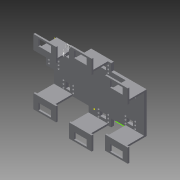
# Autodesk Inventor part: BassStuffMounts
Saved by Autodesk Inventor 2015 (Build 190159000, 159)
## iProperties
Created: 2016-04-25
Part Number: BassStuffMounts
Material: Generic
Document SubType Name: Modeling
Designer: Hatch
Density: 1 g/cm^3
Appearance: Default
Author: Hatch
Autodesk Inventor part; units mm, degrees
ref_plane "YZ Plane" through (0, 0, 0) normal (1, 0, 0) x (0, 1, 0)
ref_plane "XZ Plane" through (0, 0, 0) normal (0, 1, 0) x (-1, 0, 0)
ref_plane "XY Plane" through (0, 0, 0) normal (0, 0, 1) x (1, 0, 0)
sketch "Sketch1" plane through (0, 0, 0) normal (0, 1, 0) x (-1, 0, 0)
  line L0 (-75, 37.5) -> (75, 37.5)
  line L1 (75, 37.5) -> (75, -37.5)
  line L2 (75, -37.5) -> (-75, -37.5)
  line L3 (-75, -37.5) -> (-75, 37.5)
  line L4 (-75, 37.5) -> (75, -37.5) construction
  line L5 (75, 37.5) -> (-75, -37.5) construction
  point P0 (0, 0)
  dimension "d0" = 150
  dimension "d1" = 75
  constraints: 12 end point, 2 midpoint, 2 parallel, 1 horizontal, 1 perpendicular
  measures "d0" distance of L1.end L2.end
  measures "d1" distance of L0.end L1.end
extrude "Extrusion1" add sketch "Sketch1" along normal blind 5
sketch "Sketch2" plane through (0, 5, 0) normal (0, 1, 0) x (1, 0, 0)
  point P0 (0, 0)
sketch "Sketch3" plane through (0, 5, 0) normal (0, 1, 0) x (1, 0, 0)
  line L0 (75, 37.5) -> (-75, 37.5) projected
  line L1 (-75, 37.5) -> (-75, -37.5) projected
  line L2 (-75, 0) -> (75, 0)
  line L3 (75, -37.5) -> (75, 37.5) projected
  line L4 (-75, 0) -> (-75, -37.5)
  line L5 (-75, 0) -> (-75, 37.5)
  line L6 (-75, -18.75) -> (75, -18.75)
  line L7 (-75, 18.75) -> (75, 18.75)
  line L8 (-75, -37.5) -> (75, -37.5)
  line L9 (-75, -37.5) -> (75, -37.5) projected
  line L10 (-75, -37.5) -> (-25, -37.5)
  line L11 (-25, -37.5) -> (25, -37.5)
  line L12 (25, -37.5) -> (75, -37.5)
  line L13 (25, -37.5) -> (25, 37.5)
  line L14 (-25, -37.5) -> (-25, 37.5)
  line L15 (-75, 37.5) -> (-39, 37.5)
  line L16 (-39, 37.5) -> (-39, 13.5)
  line L17 (-39, 13.5) -> (-75, 13.5)
  line L18 (-75, 13.5) -> (-75, 37.5)
  line L19 (-75, -37.5) -> (-39, -37.5)
  line L20 (-39, -37.5) -> (-39, -13.5)
  line L21 (-39, -13.5) -> (-75, -13.5)
  line L22 (-75, -13.5) -> (-75, -37.5)
  line L23 (-67.8885, -37.5) -> (-67.8885, -31.5)
  line L24 (-70.151, 37.5) -> (-70.151, 31.5)
  line L25 (-75, -23.3322) -> (-67, -23.3322)
  circle A0 centre (-67, -31.5) radius 2.125
  line L26 (-67, -31.5) -> (-49, -31.5)
  circle A1 centre (-49, -31.5) radius 2.125
  line L27 (-67, -31.5) -> (-67, -25.5)
  line L28 (-67, -25.5) -> (-67, -19.5)
  circle A2 centre (-67, -25.5) radius 2.125
  circle A3 centre (-67, -19.5) radius 2.125
  line L29 (-49, -31.5) -> (-49, -25.5)
  line L30 (-49, -25.5) -> (-49, -19.5)
  circle A4 centre (-49, -25.5) radius 2.125
  circle A5 centre (-49, -19.5) radius 2.125
  circle A6 centre (-67, 31.5) radius 2.125
  line L31 (-67, 31.5) -> (-67, 25.5)
  line L32 (-67, 25.5) -> (-67, 19.5)
  line L33 (-67, 19.5) -> (-49, 19.5)
  line L34 (-49, 19.5) -> (-49, 25.5)
  line L35 (-49, 25.5) -> (-49, 31.5)
  circle A7 centre (-49, 31.5) radius 2.125
  circle A8 centre (-49, 25.5) radius 2.125
  circle A9 centre (-49, 19.5) radius 2.125
  circle A10 centre (-67, 25.5) radius 2.125
  circle A11 centre (-67, 19.5) radius 2.125
  point P0 (0, 0)
  dimension "d4" = 50
  dimension "d5" = 50
  dimension "d6" = 50
  dimension "d7" = 36
  dimension "d8" = 24
  dimension "d10" = 36
  dimension "d11" = 24
  dimension "d12" = 6
  dimension "d13" = 6
  dimension "d17" = 8
  dimension "d18" = 4.25
  dimension "d19" = 18
  dimension "d20" = 4.25
  dimension "d21" = 6
  dimension "d22" = 6
  dimension "d23" = 4.25
  dimension "d24" = 4.25
  dimension "d25" = 6
  dimension "d26" = 6
  dimension "d27" = 4.25
  dimension "d28" = 4.25
  dimension "d29" = 4.25
  dimension "d30" = 6
  dimension "d31" = 6
  dimension "d32" = 18
  dimension "d33" = 6
  dimension "d34" = 6
  dimension "d35" = 4.25
  dimension "d36" = 4.25
  dimension "d37" = 4.25
  dimension "d38" = 4.25
  dimension "d39" = 4.25
  constraints: 64 end point, 13 point on line, 12 centre point, 10 coincident, 10 perpendicular, 5 parallel, 4 collinear, 4 midpoint, 3 horizontal, 3 vertical
  measures "d4" distance of L1.end L10.end
  measures "d5" distance of L10.end L11.end
  measures "d6" distance of L11.end L3.start
  measures "d7" distance of L16.end L17.end
  measures "d8" distance of L15.end L16.end
  measures "d10" distance of L21.end L20.end
  measures "d11" distance of L20.end L19.end
  measures "d12" distance of L23.start L23.end
  measures "d13" distance of L24.start L24.end
  measures "d17" distance of L25.start L25.end
  measures "d18" diameter of A0
  measures "d19" distance of L26.start L26.end
  measures "d20" diameter of A1
  measures "d21" distance of L26.start L27.end
  measures "d22" distance of L27.end L28.end
  measures "d23" diameter of A2
  measures "d24" diameter of A3
  measures "d25" distance of L29.start L29.end
  measures "d26" distance of L29.end L30.end
  measures "d27" diameter of A4
  measures "d28" diameter of A5
  measures "d29" diameter of A6
  measures "d30" distance of L31.start L31.end
  measures "d31" distance of L31.end L32.end
  measures "d32" distance of L32.end L33.end
  measures "d33" distance of L33.end L34.end
  measures "d34" distance of L34.end L35.end
  measures "d35" diameter of A7
  measures "d36" diameter of A8
  measures "d37" diameter of A9
  measures "d38" diameter of A10
  measures "d39" diameter of A11
sketch "Sketch4" plane through (0, 0, 0) normal (0, -1, 0) x (1, 0, 0)
  line L0 (-75, -37.5) -> (-41, -37.5)
  line L1 (-41, -37.5) -> (-41, -34.5)
  line L2 (-41, -34.5) -> (-75, -34.5)
  line L3 (-75, -34.5) -> (-75, -37.5)
  circle A0 centre (-49, -25.5) radius 2.125 projected
  line L4 (-75, 37.5) -> (-41, 37.5)
  line L5 (-41, 37.5) -> (-41, 34.5)
  line L6 (-41, 34.5) -> (-75, 34.5)
  line L7 (-75, 34.5) -> (-75, 37.5)
  point P0 (0, 0)
  dimension "d42" = 34
  dimension "d43" = 3
  dimension "d45" = 3
  constraints: 16 end point, 4 parallel, 2 horizontal, 2 perpendicular
  measures "d42" distance of L2.end L1.end
  measures "d43" distance of L1.end L0.end
  measures "d45" distance of L4.end L5.end
extrude "Extrusion3" add sketch "Sketch4" along normal blind 34.05 contours L3 L2 L1 L0 | L4 L5 L6 L7
sketch "Sketch5" plane through (0, -34.05, 0) normal (0, -1, 0) x (1, 0, 0)
  line L0 (-75, -34.5) -> (-79, -34.5)
  line L1 (-79, -34.5) -> (-79, -37.5)
  line L2 (-79, -37.5) -> (-75, -37.5)
  line L3 (-75, -37.5) -> (-75, -34.5)
  line L4 (-41, -37.5) -> (-37, -37.5)
  line L5 (-37, -37.5) -> (-37, -34.5)
  line L6 (-37, -34.5) -> (-41, -34.5)
  line L7 (-41, -34.5) -> (-41, -37.5)
  line L8 (-75, 37.5) -> (-79, 37.5)
  line L9 (-79, 37.5) -> (-79, 34.5)
  line L10 (-79, 34.5) -> (-75, 34.5)
  line L11 (-75, 34.5) -> (-75, 37.5)
  line L12 (-41, 34.5) -> (-37, 34.5)
  line L13 (-37, 34.5) -> (-37, 37.5)
  line L14 (-37, 37.5) -> (-41, 37.5)
  line L15 (-41, 37.5) -> (-41, 34.5)
  point P0 (0, 0)
  dimension "d48" = 4
  dimension "d49" = 3
  dimension "d50" = 4
  dimension "d51" = 3
  dimension "d52" = 4
  dimension "d53" = 3
  dimension "d54" = 4
  dimension "d55" = 3
  constraints: 32 end point, 8 parallel, 4 horizontal, 4 perpendicular
  measures "d48" distance of L2.end L1.end
  measures "d49" distance of L1.end L0.end
  measures "d50" distance of L6.end L5.end
  measures "d51" distance of L5.end L4.end
  measures "d52" distance of L10.end L9.end
  measures "d53" distance of L9.end L8.end
  measures "d54" distance of L14.end L13.end
  measures "d55" distance of L13.end L12.end
extrude "Extrusion4" add sketch "Sketch5" against normal blind 3
sketch "Sketch6" plane through (-75, 5, 37.5) normal (0, 0, 1) x (1, 0, 0)
  line L0 (38, -39.05) -> (-4, -39.05)
  line L1 (-4, -39.05) -> (-4, -36.05)
  line L2 (-4, -36.05) -> (38, -36.05)
  line L3 (38, -36.05) -> (38, -39.05)
  point P0 (75, -5)
  constraints: 8 end point, 2 parallel, 1 horizontal, 1 perpendicular
extrude "Extrusion5" add sketch "Sketch6" along normal blind 23
sketch "Sketch7" plane through (75, 5, -37.5) normal (0, 0, -1) x (-1, 0, 0)
  line L0 (154, -39.05) -> (112, -39.05)
  line L1 (112, -39.05) -> (112, -36.05)
  line L2 (112, -36.05) -> (154, -36.05)
  line L3 (154, -36.05) -> (154, -39.05)
  point P0 (75, -5)
  constraints: 8 end point, 2 parallel, 1 horizontal, 1 perpendicular
extrude "Extrusion6" add sketch "Sketch7" along normal blind 23
sketch "Sketch9" plane through (0, 5, 0) normal (0, 1, 0) x (1, 0, 0)
  line L0 (-79, 60.5) -> (-37, 60.5)
  line L1 (-79, 60.5) -> (-37, 60.5) projected
  line L2 (75, 37.5) -> (-75, 37.5) projected
  line L3 (-58, 37.5) -> (-58, 31.5)
  circle A0 centre (-58, 31.5) radius 2.125
  line L4 (-58, 31.5) -> (-40, 31.5)
  line L5 (-40, 31.5) -> (-40, 25.5)
  line L6 (-40, 25.5) -> (-40, 19.5)
  circle A1 centre (-40, 31.5) radius 2.125
  circle A2 centre (-40, 25.5) radius 2.125
  circle A3 centre (-40, 19.5) radius 2.125
  circle A4 centre (-58, 25.5) radius 2.125
  circle A5 centre (-58, 19.5) radius 2.125
  line L7 (-79, -60.5) -> (-37, -60.5)
  line L8 (-79, -60.5) -> (-37, -60.5) projected
  line L9 (-75, -37.5) -> (75, -37.5) projected
  line L10 (-58, -37.5) -> (-58, -31.5)
  circle A6 centre (-58, -31.5) radius 2.125
  line L11 (-58, -31.5) -> (-40, -31.5)
  line L12 (-40, -31.5) -> (-40, -25.5)
  line L13 (-40, -25.5) -> (-40, -19.5)
  circle A7 centre (-40, -31.5) radius 2.125
  circle A8 centre (-40, -25.5) radius 2.125
  circle A9 centre (-40, -19.5) radius 2.125
  circle A10 centre (-58, -25.5) radius 2.125
  circle A11 centre (-58, -19.5) radius 2.125
  point P0 (0, 0)
  dimension "d62" = 6
  dimension "d63" = 4.25
  dimension "d64" = 18
  dimension "d65" = 6
  dimension "d66" = 6
  dimension "d67" = 4.25
  dimension "d68" = 4.25
  dimension "d69" = 4.25
  dimension "d70" = 4.25
  dimension "d71" = 4.25
  dimension "d72" = 6
  dimension "d73" = 4.25
  dimension "d74" = 18
  dimension "d75" = 6
  dimension "d76" = 6
  dimension "d77" = 4.25
  dimension "d78" = 4.25
  dimension "d79" = 4.25
  dimension "d80" = 4.25
  dimension "d81" = 4.25
  constraints: 20 end point, 12 centre point, 8 coincident, 4 horizontal, 3 point on line, 2 perpendicular, 1 vertical
  measures "d62" distance of L3.start L3.end
  measures "d63" diameter of A0
  measures "d64" distance of L4.start L4.end
  measures "d65" distance of L4.end L5.end
  measures "d66" distance of L5.end L6.end
  measures "d67" diameter of A1
  measures "d68" diameter of A2
  measures "d69" diameter of A3
  measures "d70" diameter of A4
  measures "d71" diameter of A5
  measures "d72" distance of L10.start L10.end
  measures "d73" diameter of A6
  measures "d74" distance of L11.start L11.end
  measures "d75" distance of L11.end L12.end
  measures "d76" distance of L12.end L13.end
  measures "d77" diameter of A7
  measures "d78" diameter of A8
  measures "d79" diameter of A9
  measures "d80" diameter of A10
  measures "d81" diameter of A11
extrude "Extrusion7" cut sketch "Sketch9" against normal through all
sketch "Sketch10" plane through (0, -34.05, 0) normal (0, -1, 0) x (1, 0, 0)
  line L0 (-75, -34.5) -> (-41, -34.5) projected
  line L1 (-58, -34.5) -> (-58, -45.5)
  line L2 (-41, 34.5) -> (-75, 34.5) projected
  line L3 (-58, 34.5) -> (-58, 45.5)
  line L4 (-37, -60.5) -> (-37, -34.5) projected
  line L5 (-37, -47.5) -> (-39.25, -47.5)
  line L6 (-79, -34.5) -> (-79, -60.5) projected
  line L7 (-79, -47.5) -> (-76.75, -47.5)
  line L8 (-79, -60.5) -> (-37, -60.5) projected
  line L9 (-58, -60.5) -> (-58, -57.5)
  line L10 (-46.25, -57.5) -> (-69.75, -57.5)
  line L11 (-69.75, -57.5) -> (-69.75, -45.5)
  line L12 (-69.75, -45.5) -> (-46.25, -45.5)
  line L13 (-46.25, -45.5) -> (-46.25, -57.5)
  line L14 (-79, 34.5) -> (-79, 60.5) projected
  line L15 (-79, 47.5) -> (-76.75, 47.5)
  line L16 (-37, 34.5) -> (-37, 60.5) projected
  line L17 (-37, 47.5) -> (-39.25, 47.5)
  line L18 (-37, 60.5) -> (-79, 60.5) projected
  line L19 (-58, 60.5) -> (-58, 57.5)
  line L20 (-46.25, 57.5) -> (-69.75, 57.5)
  line L21 (-69.75, 57.5) -> (-69.75, 45.5)
  line L22 (-69.75, 45.5) -> (-46.25, 45.5)
  line L23 (-46.25, 45.5) -> (-46.25, 57.5)
  point P0 (0, 0)
  dimension "d84" = 11
  dimension "d85" = 11
  dimension "d86" = 2.25
  dimension "d87" = 2.25
  dimension "d88" = 3
  dimension "d89" = 2.25
  dimension "d90" = 2.25
  dimension "d91" = 3
  dimension "d115" = 23.5
  dimension "d116" = 23.5
  constraints: 32 end point, 10 midpoint, 6 horizontal, 4 parallel, 4 vertical, 2 perpendicular
  measures "d84" distance of L1.start L1.end
  measures "d85" distance of L3.end L3.start
  measures "d86" distance of L5.start L5.end
  measures "d87" distance of L7.start L7.end
  measures "d88" distance of L9.end L9.start
  measures "d89" distance of L15.start L15.end
  measures "d90" distance of L17.start L17.end
  measures "d91" distance of L19.start L19.end
  measures "d115" distance of L10.start L10.end
  measures "d116" distance of L20.start L20.end
extrude "Extrusion8" cut sketch "Sketch10" against normal through all
sketch "Sketch14" plane through (0, 5, 0) normal (0, 1, 0) x (1, 0, 0)
  line L0 (-75, -37.5) -> (75, -37.5) projected
  line L1 (75, 37.5) -> (-32.8207, 37.5)
  line L2 (-32.8207, 37.5) -> (-32.8207, -37.5)
  line L3 (-32.8207, -37.5) -> (75, -37.5)
  line L4 (75, -37.5) -> (75, 37.5)
  point P0 (0, 0)
  constraints: 8 end point, 2 parallel, 1 horizontal, 1 perpendicular, 1 point on line
sketch "Sketch15" plane through (0, 0, 0) normal (0, -1, 0) x (1, 0, 0)
  circle A0 centre (-40, 25.5) radius 2.125 projected
  line L0 (-40, 25.5) -> (-49, 25.5)
  line L1 (-53, 20) -> (-45, 20)
  line L2 (-45, 20) -> (-45, 31)
  line L3 (-45, 31) -> (-53, 31)
  line L4 (-53, 31) -> (-53, 20)
  line L5 (-53, 20) -> (-45, 31) construction
  line L6 (-45, 20) -> (-53, 31) construction
  line L7 (-53, -31) -> (-45, -31)
  line L8 (-45, -31) -> (-45, -20)
  line L9 (-45, -20) -> (-53, -20)
  line L10 (-53, -20) -> (-53, -31)
  line L11 (-53, -31) -> (-45, -20) construction
  line L12 (-45, -31) -> (-53, -20) construction
  point P0 (0, 0)
  point P1 (-49, -25.5)
  dimension "d108" = 9
  dimension "d109" = 8
  dimension "d110" = 11
  dimension "d111" = 8
  dimension "d112" = 11
  constraints: 26 end point, 4 midpoint, 4 parallel, 3 horizontal, 2 perpendicular
  measures "d108" distance of L0.start L0.end
  measures "d109" distance of L3.end L2.end
  measures "d110" distance of L2.end L1.end
  measures "d111" distance of L9.end L8.end
  measures "d112" distance of L8.end L7.end
extrude "Extrusion13" cut sketch "Sketch15" against normal through all contours L4 L3 L2 L1 | L10 L9 L8 L7
sketch "Sketch16" plane through (0, -34.05, 0) normal (0, -1, 0) x (1, 0, 0)
  point P0 (0, 0)
sketch "Sketch18" plane through (0, 5, 0) normal (0, 1, 0) x (1, 0, 0)
  point P0 (0, 0)
sketch "Sketch19" plane through (0, 5, 0) normal (0, 1, 0) x (1, 0, 0)
  line L0 (-75, -37.5) -> (75, -37.5) projected
  line L1 (25.0535, -37.5) -> (-10.9465, -37.5)
  line L2 (-10.9465, -37.5) -> (-10.9465, -13.5)
  line L3 (-10.9465, -13.5) -> (25.0535, -13.5)
  line L4 (25.0535, -13.5) -> (25.0535, -37.5)
  line L5 (-41, 37.5) -> (75, 37.5) projected
  line L6 (25.0535, 37.5) -> (-10.9465, 37.5)
  line L7 (-10.9465, 37.5) -> (-10.9465, 13.5)
  line L8 (-10.9465, 13.5) -> (25.0535, 13.5)
  line L9 (25.0535, 13.5) -> (25.0535, 37.5)
  line L10 (-10.9465, 37.5) -> (25.0535, 37.5)
  line L11 (25.0535, 37.5) -> (25.0535, 51.5)
  line L12 (25.0535, 51.5) -> (-10.9465, 51.5)
  line L13 (-10.9465, 51.5) -> (-10.9465, 37.5)
  line L14 (-10.9465, -37.5) -> (25.0535, -37.5)
  line L15 (25.0535, -37.5) -> (25.0535, -51.5)
  line L16 (25.0535, -51.5) -> (-10.9465, -51.5)
  line L17 (-10.9465, -51.5) -> (-10.9465, -37.5)
  point P0 (0, 0)
  dimension "d117" = 36
  dimension "d118" = 24
  dimension "d119" = 36
  dimension "d120" = 24
  dimension "d121" = 14
  dimension "d122" = 14
  constraints: 32 end point, 8 parallel, 4 horizontal, 4 perpendicular, 4 point on line
  measures "d117" distance of L2.end L3.end
  measures "d118" distance of L1.end L2.end
  measures "d119" distance of L8.end L7.end
  measures "d120" distance of L7.end L6.end
  measures "d121" distance of L11.end L10.end
  measures "d122" distance of L14.end L15.end
extrude "Extrusion14" add sketch "Sketch19" against normal blind 5 contours L0 L15 L16 L17 | L13 L12 L11 L5
sketch "Sketch21" plane through (0, 0, 0) normal (0, -1, 0) x (1, 0, 0)
  line L0 (-10.9465, -37.5) -> (-10.9465, -51.5) projected
  line L1 (25.0535, -51.5) -> (-10.9465, -51.5)
  line L2 (-10.9465, -51.5) -> (-10.9465, -48.5)
  line L3 (-10.9465, -48.5) -> (25.0535, -48.5)
  line L4 (25.0535, -48.5) -> (25.0535, -51.5)
  line L5 (25.0535, 37.5) -> (25.0535, 51.5) projected
  line L6 (-10.9465, 51.5) -> (25.0535, 51.5)
  line L7 (25.0535, 51.5) -> (25.0535, 48.5)
  line L8 (25.0535, 48.5) -> (-10.9465, 48.5)
  line L9 (-10.9465, 48.5) -> (-10.9465, 51.5)
  point P0 (0, 0)
  dimension "d153" = 3
  dimension "d154" = 3
  constraints: 16 end point, 4 parallel, 2 horizontal, 2 perpendicular, 2 point on line
  measures "d153" distance of L1.end L2.end
  measures "d154" distance of L6.end L7.end
extrude "Extrusion16" add sketch "Sketch21" along normal blind 34.05
sketch "Sketch23" plane through (0, -34.05, 0) normal (0, -1, 0) x (1, 0, 0)
  line L0 (25.0535, 48.5) -> (29.0535, 48.5)
  line L1 (25.0535, -48.5) -> (29.0535, -48.5)
  line L2 (29.0535, 48.5) -> (-12.9465, 48.5)
  line L3 (-12.9465, 48.5) -> (-12.9465, 74.5)
  line L4 (-12.9465, 74.5) -> (29.0535, 74.5)
  line L5 (29.0535, 74.5) -> (29.0535, 48.5)
  line L6 (29.0535, -48.5) -> (-12.9465, -48.5)
  line L7 (-12.9465, -48.5) -> (-12.9465, -74.5)
  line L8 (-12.9465, -74.5) -> (29.0535, -74.5)
  line L9 (29.0535, -74.5) -> (29.0535, -48.5)
  point P0 (0, 0)
  dimension "d157" = 4
  dimension "d158" = 42
  dimension "d159" = 26
  dimension "d160" = 26
  constraints: 20 end point, 4 horizontal, 4 parallel, 2 perpendicular
  measures "d157" distance of L0.start L0.end
  measures "d158" distance of L3.end L4.end
  measures "d159" distance of L2.end L3.end
  measures "d160" distance of L7.end L6.end
extrude "Extrusion17" add sketch "Sketch23" against normal blind 3
sketch "Sketch24" plane through (0, 5, 0) normal (0, 1, 0) x (1, 0, 0)
  line L0 (25.0535, -37.5) -> (31.0535, -37.5)
  line L1 (31.0535, -37.5) -> (31.0535, -51.5)
  line L2 (31.0535, -51.5) -> (25.0535, -51.5)
  line L3 (25.0535, -51.5) -> (25.0535, -37.5)
  line L4 (25.0535, 51.5) -> (31.0535, 51.5)
  line L5 (31.0535, 51.5) -> (31.0535, 37.5)
  line L6 (31.0535, 37.5) -> (25.0535, 37.5)
  line L7 (25.0535, 37.5) -> (25.0535, 51.5)
  point P0 (0, 0)
  dimension "d169" = 6
  dimension "d170" = 6
  constraints: 16 end point, 4 parallel, 2 horizontal, 2 perpendicular
  measures "d169" distance of L1.end L2.end
  measures "d170" distance of L5.end L6.end
extrude "Extrusion18" add sketch "Sketch24" against normal blind 5
sketch "Sketch20" plane through (0, 5, 0) normal (0, 1, 0) x (1, 0, 0)
  line L0 (25.0535, -51.5) -> (-10.9465, -51.5) projected
  line L1 (7.0535, -51.5) -> (7.0535, -45.5)
  line L2 (7.0535, -45.5) -> (16.0535, -45.5)
  line L3 (16.0535, -45.5) -> (-1.9465, -45.5)
  line L4 (-10.9465, 51.5) -> (25.0535, 51.5) projected
  line L5 (25.0535, 51.5) -> (-10.9465, 51.5) projected
  line L6 (-6.3335, 51.5) -> (-6.3335, 45.5)
  line L7 (16.0535, -45.5) -> (16.0535, -39.5)
  line L8 (16.0535, -39.5) -> (16.0535, -33.5)
  circle A0 centre (7.0535, 39.5) radius 2.125
  circle A1 centre (7.0535, 45.5) radius 2.125
  circle A2 centre (7.0535, 33.5) radius 2.125
  circle A3 centre (7.0535, -33.5) radius 2.125
  circle A4 centre (7.0535, -39.5) radius 2.125
  circle A5 centre (7.0535, -45.5) radius 2.125
  line L9 (7.0535, -33.5) -> (25.0535, -33.5)
  circle A6 centre (25.0535, -33.5) radius 2.125
  circle A7 centre (25.0535, -39.5) radius 2.125
  circle A8 centre (25.0535, -45.5) radius 2.125
  circle A9 centre (25.0535, 45.5) radius 2.125
  circle A10 centre (25.0535, 39.5) radius 2.125
  circle A11 centre (25.0535, 33.5) radius 2.125
  line L10 (21.5535, -43.5) -> (10.5535, -43.5)
  line L11 (10.5535, -43.5) -> (10.5535, -35.5)
  line L12 (10.5535, -35.5) -> (21.5535, -35.5)
  line L13 (21.5535, -35.5) -> (21.5535, -43.5)
  line L14 (21.5535, -43.5) -> (10.5535, -35.5) construction
  line L15 (10.5535, -43.5) -> (21.5535, -35.5) construction
  line L16 (21.5535, 35.5) -> (10.5535, 35.5)
  line L17 (10.5535, 35.5) -> (10.5535, 43.5)
  line L18 (10.5535, 43.5) -> (21.5535, 43.5)
  line L19 (21.5535, 43.5) -> (21.5535, 35.5)
  line L20 (21.5535, 35.5) -> (10.5535, 43.5) construction
  line L21 (10.5535, 35.5) -> (21.5535, 43.5) construction
  point P0 (0, 0)
  point P1 (16.0535, 39.5)
  dimension "d125" = 6
  dimension "d126" = 9
  dimension "d127" = 18
  dimension "d130" = 6
  dimension "d135" = 6
  dimension "d136" = 6
  dimension "d164" = 4.25
  dimension "d165" = 4.25
  dimension "d166" = 4.25
  dimension "d167" = 4.25
  dimension "d168" = 4.25
  dimension "d173" = 4.25
  dimension "d174" = 4.25
  dimension "d175" = 4.25
  dimension "d176" = 4.25
  dimension "d177" = 4.25
  dimension "d178" = 4.25
  dimension "d179" = 11
  dimension "d180" = 8
  dimension "d181" = 11
  dimension "d182" = 8
  constraints: 38 end point, 12 centre point, 5 midpoint, 5 perpendicular, 4 coincident, 4 parallel, 4 point on line, 3 horizontal, 1 vertical
  measures "d125" distance of L1.start L1.end
  measures "d126" distance of L1.end L2.end
  measures "d127" distance of L2.end L3.end
  measures "d130" distance of L6.start L6.end
  measures "d135" distance of L2.end L7.end
  measures "d136" distance of L7.end L8.end
  measures "d164" diameter of A1
  measures "d165" diameter of A2
  measures "d166" diameter of A3
  measures "d167" diameter of A4
  measures "d168" diameter of A5
  measures "d173" diameter of A6
  measures "d174" diameter of A7
  measures "d175" diameter of A8
  measures "d176" diameter of A9
  measures "d177" diameter of A10
  measures "d178" diameter of A11
  measures "d179" distance of L11.end L12.end
  measures "d180" distance of L10.end L11.end
  measures "d181" distance of L17.end L18.end
  measures "d182" distance of L16.end L17.end
extrude "Extrusion19" cut sketch "Sketch20" against normal through all
sketch "Sketch25" plane through (0, -34.05, 0) normal (0, -1, 0) x (1, 0, 0)
  line L0 (29.0535, -74.5) -> (-12.9465, -74.5) projected
  line L1 (8.0535, -74.5) -> (8.0535, -71.5)
  line L2 (-12.9465, 74.5) -> (29.0535, 74.5) projected
  line L3 (8.0535, 74.5) -> (8.0535, 71.5)
  line L4 (8.0535, -71.5) -> (8.0535, -59.5)
  line L5 (8.0535, 71.5) -> (8.0535, 59.5)
  line L6 (19.8035, 71.5) -> (-3.6965, 71.5)
  line L7 (-3.6965, 71.5) -> (-3.6965, 59.5)
  line L8 (-3.6965, 59.5) -> (19.8035, 59.5)
  line L9 (19.8035, 59.5) -> (19.8035, 71.5)
  line L10 (19.8035, 71.5) -> (-3.6965, 59.5) construction
  line L11 (-3.6965, 71.5) -> (19.8035, 59.5) construction
  line L12 (19.8035, -59.5) -> (-3.6965, -59.5)
  line L13 (-3.6965, -59.5) -> (-3.6965, -71.5)
  line L14 (-3.6965, -71.5) -> (19.8035, -71.5)
  line L15 (19.8035, -71.5) -> (19.8035, -59.5)
  line L16 (19.8035, -59.5) -> (-3.6965, -71.5) construction
  line L17 (-3.6965, -59.5) -> (19.8035, -71.5) construction
  point P0 (0, 0)
  point P1 (8.0535, 65.5)
  point P2 (8.0535, -65.5)
  dimension "d185" = 3
  dimension "d186" = 3
  dimension "d187" = 12
  dimension "d188" = 12
  dimension "d189" = 23.5
  dimension "d190" = 23.5
  constraints: 32 end point, 8 midpoint, 4 parallel, 4 vertical, 2 horizontal, 2 perpendicular
  measures "d185" distance of L1.start L1.end
  measures "d186" distance of L3.start L3.end
  measures "d187" distance of L1.end L4.end
  measures "d188" distance of L3.end L5.end
  measures "d189" distance of L8.end L7.end
  measures "d190" distance of L14.end L13.end
extrude "Extrusion20" cut sketch "Sketch25" against normal through all
sketch "Sketch27" plane through (0, -34.05, 0) normal (0, -1, 0) x (1, 0, 0)
  line L0 (-46.25, -57.5) -> (-69.75, -57.5) projected
  line L1 (-58, -57.5) -> (8.0535, -57.5)
  line L2 (-3.6965, -59.5) -> (19.8035, -59.5) projected
  line L3 (8.0535, -57.5) -> (74.1075, -57.5)
  point P0 (0, 0)
  dimension "d193" = 66.0535
  dimension "d194" = 66.054
  constraints: 4 end point, 1 horizontal, 1 midpoint, 1 parallel
  measures "d193" distance of L1.start L1.end
  measures "d194" distance of L1.end L3.end
sketch "Sketch28" plane through (0, 0, 0) normal (0, -1, 0) x (1, 0, 0)
  circle A0 centre (-40, -31.5) radius 2.125 projected
  line L0 (75, 37.5) -> (75, -37.5) projected
  circle A1 centre (75, -31.5) radius 2.125
  line L1 (75, -31.5) -> (57, -31.5)
  circle A2 centre (57, -31.5) radius 2.125
  line L2 (57, -31.5) -> (57, -25.5)
  line L3 (57, -25.5) -> (57, -19.5)
  circle A3 centre (57, -25.5) radius 2.125
  circle A4 centre (57, -19.5) radius 2.125
  circle A5 centre (75, -25.5) radius 2.125
  circle A6 centre (75, -19.5) radius 2.125
  circle A7 centre (-40, 31.5) radius 2.125 projected
  line L4 (-40, 31.5) -> (75, 31.5)
  circle A8 centre (75, 31.5) radius 2.125
  line L5 (75, 31.5) -> (57, 31.5)
  line L6 (57, 31.5) -> (57, 25.5)
  line L7 (57, 25.5) -> (57, 19.5)
  circle A9 centre (57, 31.5) radius 2.125
  circle A10 centre (57, 25.5) radius 2.125
  circle A11 centre (57, 19.5) radius 2.125
  circle A12 centre (75, 25.5) radius 2.125
  circle A13 centre (75, 19.5) radius 2.125
  line L8 (71.5, -29.5) -> (60.5, -29.5)
  line L9 (60.5, -29.5) -> (60.5, -21.5)
  line L10 (60.5, -21.5) -> (71.5, -21.5)
  line L11 (71.5, -21.5) -> (71.5, -29.5)
  line L12 (71.5, -29.5) -> (60.5, -21.5) construction
  line L13 (60.5, -29.5) -> (71.5, -21.5) construction
  line L14 (71.5, 21.5) -> (60.5, 21.5)
  line L15 (60.5, 21.5) -> (60.5, 29.5)
  line L16 (60.5, 29.5) -> (71.5, 29.5)
  line L17 (71.5, 29.5) -> (71.5, 21.5)
  line L18 (71.5, 21.5) -> (60.5, 29.5) construction
  line L19 (60.5, 21.5) -> (71.5, 29.5) construction
  point P0 (0, 0)
  point P1 (66, -25.5)
  point P2 (66, 25.5)
  dimension "d195" = 4.25
  dimension "d196" = 18
  dimension "d197" = 4.25
  dimension "d198" = 6
  dimension "d199" = 6
  dimension "d200" = 4.25
  dimension "d201" = 4.25
  dimension "d202" = 4.25
  dimension "d203" = 4.25
  dimension "d204" = 4.25
  dimension "d205" = 6
  dimension "d206" = 6
  dimension "d207" = 4.25
  dimension "d208" = 4.25
  dimension "d209" = 4.25
  dimension "d210" = 4.25
  dimension "d211" = 4.25
  dimension "d212" = 11
  dimension "d213" = 8
  dimension "d214" = 11
  dimension "d215" = 8
  constraints: 38 end point, 12 centre point, 8 point on line, 7 coincident, 4 midpoint, 4 parallel, 4 perpendicular, 3 horizontal, 1 vertical
  measures "d195" diameter of A1
  measures "d196" distance of L1.start L1.end
  measures "d197" diameter of A2
  measures "d198" distance of L2.start L2.end
  measures "d199" distance of L2.end L3.end
  measures "d200" diameter of A3
  measures "d201" diameter of A4
  measures "d202" diameter of A5
  measures "d203" diameter of A6
  measures "d204" diameter of A8
  measures "d205" distance of L5.end L6.end
  measures "d206" distance of L6.end L7.end
  measures "d207" diameter of A9
  measures "d208" diameter of A10
  measures "d209" diameter of A11
  measures "d210" diameter of A12
  measures "d211" diameter of A13
  measures "d212" distance of L9.end L10.end
  measures "d213" distance of L8.end L9.end
  measures "d214" distance of L15.end L16.end
  measures "d215" distance of L14.end L15.end
sketch "Sketch29" plane through (75, 0, 37.5) normal (1, 0, 0) x (0, 0, -1)
  line L0 (75, 0) -> (0, 0)
  line L1 (0, 0) -> (0, 5)
  line L2 (0, 5) -> (75, 5)
  line L3 (75, 5) -> (75, 0)
  point P0 (37.5, 0)
  constraints: 8 end point, 2 parallel, 1 horizontal, 1 perpendicular
extrude "Extrusion21" add sketch "Sketch29" along normal blind 5
extrude "Extrusion22" cut sketch "Sketch28" against normal through all contours A8 L0 | L0 L4 A8 | L0 A8 L4 | A12 L0 | L0 A12 | A13 L0 | L0 A13 | A6 L0 | L0 A6 | A5 L0 | L0 A5 | A1 L0 | L0 L1 A1 | L0 A1 L1 | A2 L2 L1 | L1 L2 A2 | A3 L3 L2 | L2 L3 A3 | A4 | L4 A9 | L6 A9 L4 | L4 A9 L6 | A10 L7 L6 | L6 L7 A10 | A11 | L8 L9 L10 L11 | L14 L15 L16 L17
sketch "Sketch30" plane through (0, 0, 0) normal (0, -1, 0) x (1, 0, 0)
  line L0 (31.0535, -37.5) -> (80, -37.5) projected
  line L1 (75, -37.5) -> (58, -37.5)
  line L2 (58, -37.5) -> (58, -34.5)
  line L3 (58, -34.5) -> (75, -34.5)
  line L4 (75, -34.5) -> (75, -37.5)
  line L5 (75, -34.5) -> (92, -34.5)
  line L6 (92, -34.5) -> (92, -37.5)
  line L7 (92, -37.5) -> (75, -37.5)
  line L8 (75, -37.5) -> (75, -34.5)
  line L9 (80, 37.5) -> (31.0535, 37.5) projected
  line L10 (58, 37.5) -> (92, 37.5)
  line L11 (92, 37.5) -> (92, 34.5)
  line L12 (92, 34.5) -> (58, 34.5)
  line L13 (58, 34.5) -> (58, 37.5)
  point P0 (0, 0)
  dimension "d220" = 17
  dimension "d221" = 3
  dimension "d222" = 17
  dimension "d223" = 3
  constraints: 24 end point, 6 parallel, 5 point on line, 3 horizontal, 3 perpendicular
  measures "d220" distance of L2.end L3.end
  measures "d221" distance of L1.end L2.end
  measures "d222" distance of L6.end L7.end
  measures "d223" distance of L10.end L11.end
extrude "Extrusion23" add sketch "Sketch30" along normal blind 34.05
sketch "Sketch31" plane through (0, -34.05, 0) normal (0, -1, 0) x (1, 0, 0)
  line L0 (58, -34.5) -> (54, -34.5)
  line L1 (54, -34.5) -> (96, -34.5)
  line L2 (96, -34.5) -> (96, -60.5)
  line L3 (96, -60.5) -> (54, -60.5)
  line L4 (54, -60.5) -> (54, -34.5)
  line L5 (54, 34.5) -> (96, 34.5)
  line L6 (96, 34.5) -> (96, 60.5)
  line L7 (96, 60.5) -> (54, 60.5)
  line L8 (54, 60.5) -> (54, 34.5)
  point P0 (0, 0)
  dimension "d226" = 4
  dimension "d227" = 42
  dimension "d228" = 26
  dimension "d229" = 42
  dimension "d230" = 26
  constraints: 18 end point, 4 parallel, 3 horizontal, 2 perpendicular
  measures "d226" distance of L0.start L0.end
  measures "d227" distance of L2.end L3.end
  measures "d228" distance of L1.end L2.end
  measures "d229" distance of L7.end L6.end
  measures "d230" distance of L6.end L5.end
extrude "Extrusion24" add sketch "Sketch31" against normal blind 3
sketch "Sketch32" plane through (0, -34.05, 0) normal (0, -1, 0) x (1, 0, 0)
  line L0 (96, -60.5) -> (54, -60.5) projected
  line L1 (75, -60.5) -> (75, -57.5)
  line L2 (75, -57.5) -> (75, -45.5)
  line L3 (54, 60.5) -> (96, 60.5) projected
  line L4 (75, 60.5) -> (75, 57.5)
  line L5 (75, 57.5) -> (75, 45.5)
  line L6 (86.75, -57.5) -> (63.25, -57.5)
  line L7 (63.25, -57.5) -> (63.25, -45.5)
  line L8 (63.25, -45.5) -> (86.75, -45.5)
  line L9 (86.75, -45.5) -> (86.75, -57.5)
  line L10 (86.75, -57.5) -> (63.25, -45.5) construction
  line L11 (63.25, -57.5) -> (86.75, -45.5) construction
  line L12 (86.75, 45.5) -> (63.25, 45.5)
  line L13 (63.25, 45.5) -> (63.25, 57.5)
  line L14 (63.25, 57.5) -> (86.75, 57.5)
  line L15 (86.75, 57.5) -> (86.75, 45.5)
  line L16 (86.75, 45.5) -> (63.25, 57.5) construction
  line L17 (63.25, 45.5) -> (86.75, 57.5) construction
  point P0 (0, 0)
  point P1 (75, -51.5)
  point P2 (75, 51.5)
  dimension "d233" = 3
  dimension "d234" = 12
  dimension "d235" = 3
  dimension "d236" = 12
  dimension "d237" = 23.5
  dimension "d238" = 23.5
  constraints: 32 end point, 8 midpoint, 4 parallel, 2 horizontal, 2 perpendicular, 2 point on line, 2 vertical
  measures "d233" distance of L1.start L1.end
  measures "d234" distance of L1.end L2.end
  measures "d235" distance of L4.start L4.end
  measures "d236" distance of L4.end L5.end
  measures "d237" distance of L7.end L8.end
  measures "d238" distance of L13.end L14.end
extrude "Extrusion25" cut sketch "Sketch32" against normal through all
sketch "Sketch33" plane through (80, 0, 37.5) normal (1, 0, 0) x (0, 0, -1)
  line L0 (0, 5) -> (75, 5)
  line L1 (75, 5) -> (75, 0)
  line L2 (75, 0) -> (0, 0)
  line L3 (0, 0) -> (0, 5)
  point P0 (37.5, 0)
  constraints: 8 end point, 2 parallel, 1 horizontal, 1 perpendicular
extrude "Extrusion26" add sketch "Sketch33" along normal blind 12
sketch "Sketch34" plane through (-75, 5, -37.5) normal (-1, 0, 0) x (0, 0, 1)
  line L0 (20.125, -5) -> (15.875, -5) projected
  line L1 (72, -5) -> (3, -5) projected
  line L2 (49.5, 0) -> (25.5, 0)
  line L3 (25.5, 0) -> (25.5, -5)
  line L4 (25.5, -5) -> (49.5, -5)
  line L5 (49.5, -5) -> (49.5, 0)
  line L6 (49.5, 0) -> (25.5, -5) construction
  line L7 (25.5, 0) -> (49.5, -5) construction
  point P0 (37.5, -5)
  point P1 (37.5, -2.5)
  dimension "d244" = 24
  constraints: 12 end point, 2 midpoint, 2 parallel, 1 horizontal, 1 perpendicular, 1 point on line
  measures "d244" distance of L4.end L3.end
extrude "Extrusion27" add sketch "Sketch34" along normal blind 36
sketch "Sketch35" plane through (0, 5, 0) normal (0, 1, 0) x (1, 0, 0)
  point P0 (0, 0)
sketch "Sketch36" plane through (0, 5, 0) normal (0, 1, 0) x (1, 0, 0)
  line L0 (-111, -12) -> (-75, -12)
  line L1 (-75, -12) -> (-93, -12)
  line L2 (-93, -12) -> (-93, 12)
  circle A0 centre (-58, -19.5) radius 2.125 projected
  line L3 (-58, -19.5) -> (-67, -19.5)
  line L4 (-67, -19.5) -> (-67, 12)
  line L5 (-93, 0) -> (-59.5316, 0)
  circle A1 centre (-67, 0) radius 2.125
  point P0 (0, 0)
  dimension "d247" = 9
  dimension "d248" = 4.25
  constraints: 12 end point, 3 horizontal, 2 midpoint, 2 point on line, 1 centre point, 1 perpendicular, 1 vertical
  measures "d247" distance of L3.start L3.end
  measures "d248" diameter of A1
extrude "Extrusion28" cut sketch "Sketch36" against normal through all contours A1 L5 L4 | L4 L5 A1 | L5 A1 L4 | L4 A1 L5
pattern_linear "Rectangular Pattern1" count 3 spacing 6 along (0, 0, 1) count 2 spacing 18 along (-1, 0, 0) of "Extrusion28" first direction both ways yes
sketch "Sketch37" plane through (0, 5, 0) normal (0, 1, 0) x (1, 0, 0)
  circle A0 centre (-85, -6) radius 2.125 projected
  line L0 (-85, -6) -> (-90, -6)
  line L1 (-111, -12) -> (-90, -12)
  line L2 (-90, -12) -> (-90, 12)
  line L3 (-90, 12) -> (-111, 12)
  line L4 (-111, 12) -> (-111, -12)
  point P0 (0, 0)
  dimension "d257" = 5
  constraints: 10 end point, 2 horizontal, 2 parallel, 1 perpendicular
  measures "d257" distance of L0.start L0.end
extrude "Extrusion29" cut sketch "Sketch37" against normal through all contours L4 L3 L2 L1
sketch "Sketch38" plane through (0, 5, 0) normal (0, 1, 0) x (1, 0, 0)
  point P0 (0, 0)
sketch "Sketch39" plane through (0, 5, 0) normal (0, 1, 0) x (1, 0, 0)
  line L0 (-79, -34.5) -> (-37, -34.5) projected
  circle A0 centre (-58, -31.5) radius 2.125 projected
  line L1 (-58, -34.5) -> (-58, -31.5)
  circle A1 centre (-58, -19.5) radius 2.125 projected
  line L2 (-58, -19.5) -> (-58, -16.5)
  circle A2 centre (-58, -25.5) radius 2.125 projected
  line L3 (-58, -25.5) -> (-49, -25.5)
  point P0 (0, 0)
  dimension "d260" = 3
  dimension "d261" = 3
  constraints: 6 end point, 2 vertical, 1 horizontal, 1 midpoint
  measures "d260" distance of L1.start L1.end
  measures "d261" distance of L2.start L2.end
sketch "Sketch40" plane through (31.0535, 0, -37.5) normal (0, 0, -1) x (-1, 0, 0)
  line L0 (-26.935, 0) -> (-8.0936, 0)
  line L1 (-8.0936, 0) -> (-8.0936, 11.7017)
  line L2 (-8.0936, 11.7017) -> (-26.935, 11.7017)
  line L3 (-26.935, 11.7017) -> (-26.935, 0)
  point P0 (31.0535, 0)
  constraints: 8 end point, 2 parallel, 1 horizontal, 1 perpendicular
body "Solid1"
